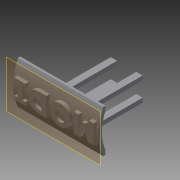
# Autodesk Inventor part: SoporteFio
Saved by Autodesk Inventor 2013 (Build 170138000, 138)
## iProperties
Created: 2013-05-06
Part Number: SoporteFio
Material: Generic
Document SubType Name: Modeling
Designer: otrab
Density: 1 g/cm^3
Author: otrab
Autodesk Inventor part; units mm, degrees
ref_plane "YZ Plane" through (0, 0, 0) normal (1, 0, 0) x (0, 1, 0)
ref_plane "XY Plane" through (0, 0, 0) normal (0, 0, 1) x (1, 0, 0)
sketch "Sketch1" plane through (0, 0, 0) normal (0, 1, 0) x (-1, 0, 0)
  line L0 (-7.5, -5.5) -> (7.5, -5.5)
  line L1 (7.5, -5.5) -> (7.5, 5.5)
  line L2 (7.5, 5.5) -> (-7.5, 5.5)
  line L3 (-7.5, 5.5) -> (-7.5, -5.5)
  line L4 (-7.5, -5.5) -> (7.5, 5.5) construction
  line L5 (7.5, -5.5) -> (-7.5, 5.5) construction
  point P0 (0, 0)
  dimension "d0" = 15
  dimension "d1" = 11
  constraints: 12 end point, 2 midpoint, 2 parallel, 1 horizontal, 1 perpendicular
  measures "d0" distance of L2.end L1.end
  measures "d1" distance of L0.end L1.end
extrude "Extrusion1" add sketch "Sketch1" along normal blind 30
sketch "Sketch2" plane through (0, 30, 0) normal (0, 1, 0) x (1, 0, 0)
  line L0 (7.5, 5.5) -> (-7.5, 5.5) projected
  line L1 (7.5, -3.5) -> (-7.5, -3.5)
  line L2 (-7.5, -3.5) -> (-7.5, 3.5)
  line L3 (-7.5, 3.5) -> (7.5, 3.5)
  line L4 (7.5, 3.5) -> (7.5, -3.5)
  line L5 (7.5, -3.5) -> (-7.5, 3.5) construction
  line L6 (-7.5, -3.5) -> (7.5, 3.5) construction
  line L7 (-7.5, 5.5) -> (-7.5, -5.5) projected
  line L8 (4.5, -5.5) -> (-4.5, -5.5)
  line L9 (-4.5, -5.5) -> (-4.5, 5.5)
  line L10 (-4.5, 5.5) -> (4.5, 5.5)
  line L11 (4.5, 5.5) -> (4.5, -5.5)
  line L12 (4.5, -5.5) -> (-4.5, 5.5) construction
  line L13 (-4.5, -5.5) -> (4.5, 5.5) construction
  point P0 (0, 0)
  dimension "d4" = 15
  dimension "d5" = 2
  dimension "d8" = 3
  constraints: 24 end point, 4 midpoint, 4 parallel, 2 horizontal, 2 perpendicular, 1 point on line
  measures "d4" distance of L2.end L3.end
  measures "d5" distance between parallel lines of L0 L3
  measures "d8" distance between parallel lines of L7 L9
extrude "Extrusion2" cut sketch "Sketch2" against normal blind 28 contours L11 L3 L9 L0 | L11 L1 L9 L3 | L3 L4 L1 L11 | L9 L1 L2 L3 | L11 L8 L9 L1
sketch "Sketch3" plane through (7.5, 0, 5.5) normal (1, 0, 0) x (0, 0, -1)
  line L0 (2, 2) -> (2, 30) projected
  line L1 (0, 30) -> (2, 30) projected
  line L2 (1, 30) -> (2, 30) construction
  line L3 (1.5, 30) -> (2, 27.042)
  line L4 (2, 27.042) -> (2, 30)
  line L5 (1.5, 30) -> (2, 30)
  point P0 (5.5, 0)
  dimension "d9" = 3
  constraints: 8 end point, 2 collinear, 2 midpoint, 1 perpendicular, 1 point on line
  measures "d9" distance of L3.start L3.end
extrude "Extrusion3" cut sketch "Sketch3" against normal through all
sketch "Sketch4" plane through (0, 0, 0) normal (0, -1, 0) x (1, 0, 0)
  line L0 (7.5, -5.5) -> (-7.5, -5.5) projected
  line L1 (-7.5, -5.5) -> (-7.5, 5.5) projected
  line L2 (0, -5.5) -> (-20, -5.5)
  line L3 (-20, -5.5) -> (-20, 14.5)
  line L4 (-20, 14.5) -> (20, 14.5)
  line L5 (20, 14.5) -> (20, -5.5)
  line L6 (20, -5.5) -> (0, -5.5)
  point P0 (0, 0)
  dimension "d12" = 20
  dimension "d13" = 20
  dimension "d14" = 40
  constraints: 10 end point, 2 parallel, 2 perpendicular, 1 collinear, 1 midpoint
  measures "d12" distance of L2.start L2.end
  measures "d13" distance of L2.end L3.end
  measures "d14" distance of L3.end L4.end
extrude "Extrusion4" add sketch "Sketch4" along normal blind 1
sketch "Sketch5" plane through (-20, 0, -5.5) normal (-1, 0, 0) x (0, 0, 1)
  line L0 (20, -1) -> (0, -1) projected
  arc A0 (0, -1) -> (20, -1) centre (10, 19.4933) ccw
  point P0 (5.5, 0)
  constraints: 2 point on circle, 1 centre point
extrude "Extrusion5" add sketch "Sketch5" against normal up to surface (40 mm away)
ref_plane "Work Plane1" through (0, -4.5, 0) normal (0, -1, 0) x (1, 0, 0)
sketch "Sketch6" plane through (0, -4.5, 0) normal (0, -1, 0) x (1, 0, 0)
  line L0 (20.1926, -0.1233) -> (-18.6074, -0.1233) construction
  line L1 (-18.6074, -0.1233) -> (-18.6074, 10.9579) construction
  line L2 (-18.6074, 10.9579) -> (20.1926, 10.9579) construction
  line L3 (20.1926, 10.9579) -> (20.1926, -0.1233) construction
  line L4 (9.6056, 9.0677) -> (11.9126, 9.0677)
  line L5 (11.9126, 9.0677) -> (11.9126, 3.0432)
  line L6 (11.9126, 3.0432) -> (13.5803, 6.9518)
  line L7 (13.5803, 6.9518) -> (15.1893, 6.9518)
  line L8 (15.1893, 6.9518) -> (16.8571, 3.0432)
  line L9 (16.8571, 3.0432) -> (16.8571, 9.0677)
  line L10 (16.8571, 9.0677) -> (19.0464, 9.0677)
  line L11 (19.0464, 9.0677) -> (19.0464, 0.0677)
  line L12 (19.0464, 0.0677) -> (16.3501, 0.0677)
  line L13 (16.3501, 0.0677) -> (14.3224, 4.586)
  line L14 (14.3224, 4.586) -> (12.302, 0.0677)
  line L15 (12.302, 0.0677) -> (9.6056, 0.0677)
  line L16 (9.6056, 0.0677) -> (9.6056, 9.0677)
  spline S0 degree 2 poles (-1.4368, 4.5713) (-1.4368, 6.724) (1.0244, 9.2587) (3.1991, 9.2587) knots 0 0 0 1 2 2 2
  spline S1 degree 2 poles (3.1991, 9.2587) (5.3738, 9.2587) (7.835, 6.724) (7.835, 4.5713) knots 0 0 0 1 2 2 2
  spline S2 degree 2 poles (7.835, 4.5713) (7.835, 2.3966) (5.3738, -0.1233) (3.1991, -0.1233) knots 0 0 0 1 2 2 2
  spline S3 degree 2 poles (3.1991, -0.1233) (1.0391, -0.1233) (-1.4368, 2.3966) (-1.4368, 4.5713) knots 0 0 0 1 2 2 2
  spline S4 degree 2 poles (1.6342, 6.8562) (1.2962, 6.4448) (0.973, 5.3207) (0.973, 4.564) knots 0 0 0 1 2 2 2
  spline S5 degree 2 poles (0.973, 4.564) (0.973, 3.7558) (1.3477, 2.6171) (1.6489, 2.2644) knots 0 0 0 1 2 2 2
  spline S6 degree 2 poles (1.6489, 2.2644) (1.9575, 1.8971) (2.7583, 1.5738) (3.1991, 1.5738) knots 0 0 0 1 2 2 2
  spline S7 degree 2 poles (3.1991, 1.5738) (3.6399, 1.5738) (4.4187, 1.8897) (4.742, 2.2497) knots 0 0 0 1 2 2 2
  spline S8 degree 2 poles (4.742, 2.2497) (5.0432, 2.5877) (5.4252, 3.7852) (5.4252, 4.5713) knots 0 0 0 1 2 2 2
  spline S9 degree 2 poles (5.4252, 4.5713) (5.4252, 5.3795) (5.0579, 6.5109) (4.7567, 6.8636) knots 0 0 0 1 2 2 2
  spline S10 degree 2 poles (4.7567, 6.8636) (4.4554, 7.2236) (3.6399, 7.5615) (3.1991, 7.5615) knots 0 0 0 1 2 2 2
  spline S11 degree 2 poles (3.1991, 7.5615) (2.7509, 7.5615) (1.9428, 7.2162) (1.6342, 6.8562) knots 0 0 0 1 2 2 2
  spline S12 degree 2 poles (-11.7152, 4.5787) (-11.7152, 5.835) (-10.5691, 7.826) (-9.6874, 8.355) knots 0 0 0 1 2 2 2
  spline S13 degree 2 poles (-9.6874, 8.355) (-9.0336, 8.7518) (-7.4613, 9.0677) (-6.3813, 9.0677) knots 0 0 0 1 2 2 2
  line L17 (-6.3813, 9.0677) -> (-3.2074, 9.0677)
  line L18 (-3.2074, 9.0677) -> (-3.2074, 0.0677)
  line L19 (-3.2074, 0.0677) -> (-6.4695, 0.0677)
  spline S14 degree 2 poles (-6.4695, 0.0677) (-7.5715, 0.0677) (-9.1731, 0.435) (-9.7168, 0.773) knots 0 0 0 1 2 2 2
  spline S15 degree 2 poles (-9.7168, 0.773) (-10.6425, 1.346) (-11.7152, 3.2709) (-11.7152, 4.5787) knots 0 0 0 1 2 2 2
  spline S16 degree 2 poles (-9.3127, 4.5566) (-9.3127, 3.6677) (-8.6662, 2.4113) (-7.9682, 2.0513) knots 0 0 0 1 2 2 2
  spline S17 degree 2 poles (-7.9682, 2.0513) (-7.6082, 1.875) (-6.8662, 1.7501) (-6.1168, 1.7501) knots 0 0 0 1 2 2 2
  line L20 (-6.1168, 1.7501) -> (-5.5291, 1.7501)
  line L21 (-5.5291, 1.7501) -> (-5.5291, 7.3779)
  line L22 (-5.5291, 7.3779) -> (-6.1168, 7.3779)
  spline S18 degree 2 poles (-6.1168, 7.3779) (-6.947, 7.3779) (-7.7184, 7.2236) (-8.0858, 7.0252) knots 0 0 0 1 2 2 2
  spline S19 degree 2 poles (-8.0858, 7.0252) (-8.7176, 6.6652) (-9.3127, 5.453) (-9.3127, 4.5566) knots 0 0 0 1 2 2 2
  line L23 (-18.3568, 9.0677) -> (-13.0817, 9.0677)
  line L24 (-13.0817, 9.0677) -> (-13.0817, 7.4734)
  line L25 (-13.0817, 7.4734) -> (-14.5584, 7.4734)
  line L26 (-14.5584, 7.4734) -> (-14.5584, 1.662)
  line L27 (-14.5584, 1.662) -> (-13.0817, 1.662)
  line L28 (-13.0817, 1.662) -> (-13.0817, 0.0677)
  line L29 (-13.0817, 0.0677) -> (-18.3568, 0.0677)
  line L30 (-18.3568, 0.0677) -> (-18.3568, 1.662)
  line L31 (-18.3568, 1.662) -> (-16.8801, 1.662)
  line L32 (-16.8801, 1.662) -> (-16.8801, 7.4734)
  line L33 (-16.8801, 7.4734) -> (-18.3568, 7.4734)
  line L34 (-18.3568, 7.4734) -> (-18.3568, 9.0677)
  point P0 (0, 0)
  constraints: 2 other
extrude "Extrusion6" add sketch "Sketch6" against normal up to surface
sketch "Sketch7" plane through (0, 2, 0) normal (0, 1, 0) x (1, 0, 0)
  line L0 (-4.5, 3.5) -> (4.5, 3.5)
  line L1 (4.5, 3.5) -> (4.5, -3.5)
  line L2 (4.5, -3.5) -> (-4.5, -3.5)
  line L3 (-4.5, -3.5) -> (-4.5, 3.5)
  line L4 (-4.5, 5.5) -> (4.5, 5.5)
  line L5 (4.5, 5.5) -> (4.5, 3.5)
  line L6 (4.5, 3.5) -> (-4.5, 3.5)
  line L7 (-4.5, 3.5) -> (-4.5, 5.5)
  line L8 (4.5, 3.5) -> (7.5, 3.5)
  line L9 (7.5, 3.5) -> (7.5, -3.5)
  line L10 (7.5, -3.5) -> (4.5, -3.5)
  line L11 (4.5, -3.5) -> (4.5, 3.5)
  line L12 (-4.5, -3.5) -> (4.5, -3.5)
  line L13 (4.5, -3.5) -> (4.5, -5.5)
  line L14 (4.5, -5.5) -> (-4.5, -5.5)
  line L15 (-4.5, -5.5) -> (-4.5, -3.5)
  line L16 (-7.5, 3.5) -> (-4.5, 3.5)
  line L17 (-4.5, 3.5) -> (-4.5, -3.5)
  line L18 (-4.5, -3.5) -> (-7.5, -3.5)
  line L19 (-7.5, -3.5) -> (-7.5, 3.5)
  point P0 (0, 0)
  constraints: 40 end point, 10 parallel, 5 horizontal, 5 perpendicular
extrude "Extrusion7" cut sketch "Sketch7" against normal blind 2
sketch "Sketch8" plane through (-20, 0, -5.5) normal (-1, 0, 0) x (0, 0, 1)
  line L0 (20, 0) -> (0, 0) projected
  arc A0 (2.0573, 0) -> (18.0573, 0) centre (10.0573, 18.6647) ccw
  point P0 (5.5, 0)
  dimension "d24" = 16
  constraints: 2 point on circle, 2 point on line, 1 centre point
  measures "d24" distance of A0.start A0.end
extrude "Extrusion8" cut sketch "Sketch8" against normal up to surface (40 mm away)
sketch "Sketch9" plane through (-7.5, 0, 3.5) normal (0, -1, 0) x (1, 0, 0)
  line L0 (0, 0) -> (0, 2) projected
  line L1 (3, 0) -> (0, 0) projected
  line L2 (0, 2) -> (3, 2)
  line L3 (3, 2) -> (3, 0)
  line L4 (3, 0) -> (0, 0)
  line L5 (0, 0) -> (0, 2)
  line L6 (12.0066, 2) -> (14.998, 2)
  line L7 (14.998, 2) -> (14.998, 0)
  line L8 (14.998, 0) -> (12.0066, 0)
  line L9 (12.0066, 0) -> (12.0066, 2)
  point P0 (7.5, -3.5)
  constraints: 16 end point, 4 parallel, 2 horizontal, 2 perpendicular
extrude "Extrusion9" add sketch "Sketch9" along normal up to surface
body "Solid1"
